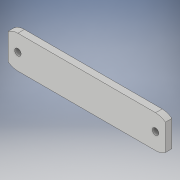
# Autodesk Inventor part: piezaboton
Saved by Autodesk Inventor 2019 (Build 230136000, 136)
## iProperties
Created: 2019-03-07
Part Number: piezaboton
Material: Genérico
Document SubType Name: Modeling
Designer: flakt
Density: 1 g/cm^3
Appearance: Valor por defecto
Author: flakt
Autodesk Inventor part; units mm, degrees
ref_plane "YZ Plane" through (0, 0, 0) normal (1, 0, 0) x (0, 1, 0)
ref_plane "XZ Plane" through (0, 0, 0) normal (0, 1, 0) x (-1, 0, 0)
ref_plane "XY Plane" through (0, 0, 0) normal (0, 0, 1) x (1, 0, 0)
sketch "Boceto1" plane through (0, 0, 0) normal (0, 0, 1) x (1, 0, 0)
  circle A0 centre (0, 0) radius 1.5
  line L0 (0, 0) -> (63, 0)
  circle A1 centre (63, 0) radius 1.5
  line L1 (0, 0) -> (0, 7.5)
  circle A2 centre (0, 0) radius 7.5
  line L2 (31.5, 0) -> (31.5, 8.9606)
  circle A3 centre (63, 0) radius 7.5
  line L3 (0, 7.5) -> (63, 7.5)
  line L4 (0, -7.5) -> (63, -7.5)
  dimension "d0" = 3
  dimension "d1" = 63
  dimension "d2" = 3
  dimension "d4" = 7.5
  constraints: 10 end point, 4 centre point, 4 point on circle, 3 coincident, 2 tangent, 2 vertical, 1 horizontal, 1 midpoint, 1 symmetric about line, 1 other
  measures "d0" diameter of A0
  measures "d1" distance of L0.start L0.end
  measures "d2" diameter of A1
  measures "d4" distance of L0.start L1.end
extrude "Extrusión1" add sketch "Boceto1" along normal blind 3 contours L0 A2 L1 A0 | A0 L1 A2 L0 | A2 L3 L2 L0 | L0 A3 L4 A2 | L2 L3 A3 L0 | A3
sketch "Boceto2" plane through (0, 0, 3) normal (0, 0, 1) x (1, 0, 0)
  arc A0 (63, -7.5) -> (63, 7.5) centre (63, 0) ccw projected
  line L0 (70.5, 0) -> (67.5, 0)
  line L1 (67.5, 8.7758) -> (71.624, 8.7758)
  line L2 (71.624, 8.7758) -> (71.624, -9.0802)
  line L3 (71.624, -9.0802) -> (67.5, -9.0802)
  line L4 (67.5, -9.0802) -> (67.5, 8.7758)
  line L5 (63, 7.5) -> (0, 7.5) projected
  line L6 (31.5, 7.5) -> (31.5, 16.2706)
  arc A1 (0, 7.5) -> (0, -7.5) centre (0, 0) ccw
  line L7 (-7.5, 0) -> (-4.5, 0)
  line L8 (-4.5, 8.7758) -> (-8.624, 8.7758)
  line L9 (-8.624, 8.7758) -> (-8.624, -9.0802)
  line L10 (-8.624, -9.0802) -> (-4.5, -9.0802)
  line L11 (-4.5, -9.0802) -> (-4.5, 8.7758)
  point P0 (0, 0)
  dimension "d7" = 3
  constraints: 22 end point, 8 symmetric about line, 4 point on circle, 2 horizontal, 2 parallel, 1 centre point, 1 midpoint, 1 perpendicular, 1 vertical, 1 other
  measures "d7" distance of L0.start L0.end
extrude "Extrusión2" cut sketch "Boceto2" against normal blind 3
